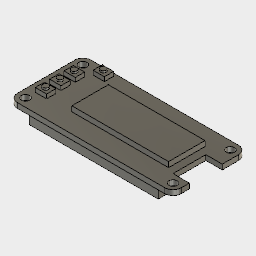
2900 Feather OLED Wing (Autodesk Fusion 360 design; units mm, degrees)
Autodesk Fusion 360 part; units mm, degrees
sketch "PCB" plane through (0, 0, 0) normal (0, 0, 1) x (1, 0, 0)
  line L0 (0, 0) -> (50.8, 0)
  line L1 (50.8, 0) -> (50.8, 22.86)
  line L2 (50.8, 22.86) -> (0, 22.86)
  line L3 (0, 22.86) -> (0, 0)
  circle A0 centre (2.54, 2.54) radius 1.27
  line L4 (0, 11.43) -> (51, 11.43) construction
  circle A1 centre (2.54, 20.32) radius 1.27
  line L5 (25.4, 22.86) -> (25.4, 0) construction
  circle A2 centre (48.26, 20.32) radius 1.27
  circle A3 centre (48.26, 2.54) radius 1.27
  line L6 (45.72, 15.24) -> (50.8, 15.24)
  line L7 (50.8, 15.24) -> (50.8, 5.08)
  line L8 (50.8, 5.08) -> (45.72, 5.08)
  line L9 (45.72, 5.08) -> (45.72, 15.24)
  dimension "d1" = 50.8
  dimension "d2" = 22.86
  dimension "d3" = 2.54
  dimension "d4" = 2.54
  dimension "d5" = 2.54
  dimension "d9" = 5.08
  dimension "d10" = 10.16
  dimension "d11" = 5.08
  measures "d1" distance of L0.start L0.end
  measures "d2" distance of L0.start L2.end
  measures "d3" diameter of A0
  measures "d4" distance of L0 A0.centre
  measures "d5" distance of L3 A0.centre
  measures "d9" distance of L6.start L6.end
  measures "d10" distance of L6.start L8.end
  measures "d11" distance of L0 L8
extrude "Extrude1" add sketch "PCB" against normal blind 1.6 contours L0 L1 L2 L3 L6 L8 L9 makes body 1
fillet "Fillet1" radius 2.54 4 edges at (0, 22.86, -0.8) (0, 0, -0.8) (50.8, 0, -0.8) (50.8, 22.86, -0.8) on bodies 1
sketch "OLED" plane through (0, 0, 0) normal (0, 0, 1) x (-1, 0, 0)
  circle A0 centre (-2.54, -2.54) radius 1.27
  circle A1 centre (-2.54, -20.32) radius 1.27
  circle A2 centre (-48.26, -2.54) radius 1.27
  circle A3 centre (-48.26, -20.32) radius 1.27
  arc A4 (-50.8, -20.32) -> (-48.26, -22.86) centre (-48.26, -20.32) ccw
  line L0 (-48.26, -22.86) -> (-2.54, -22.86)
  arc A5 (-2.54, -22.86) -> (0, -20.32) centre (-2.54, -20.32) ccw
  line L1 (0, -20.32) -> (0, -2.54)
  arc A6 (0, -2.54) -> (-2.54, 0) centre (-2.54, -2.54) ccw
  line L2 (-2.54, 0) -> (-48.26, 0)
  arc A7 (-48.26, 0) -> (-50.8, -2.54) centre (-48.26, -2.54) ccw
  line L3 (-50.8, -2.54) -> (-50.8, -5.08)
  line L4 (-50.8, -5.08) -> (-45.72, -5.08)
  line L5 (-45.72, -5.08) -> (-45.72, -15.24)
  line L6 (-45.72, -15.24) -> (-50.8, -15.24)
  line L7 (-50.8, -15.24) -> (-50.8, -20.32)
  line L8 (-13.46, -17.27) -> (-43.43, -17.27)
  line L9 (-43.43, -17.27) -> (-43.43, -5.97)
  line L10 (-43.43, -5.97) -> (-13.46, -5.97)
  line L11 (-13.46, -5.97) -> (-13.46, -17.27)
  dimension "d12" = 29.97
  dimension "d13" = 11.3
  dimension "d14" = 5.97
  dimension "d15" = 13.46
  measures "d12" distance of L9.end L10.end
  measures "d13" distance of L8.start L10.end
  measures "d14" distance of L2 L10
  measures "d15" distance of L1 L11
extrude "Extrude2" add sketch "OLED" along normal blind 1.62 separate body contours L8 L9 L10 L11 makes body 2
sketch "buttons" plane through (0, 0, 0) normal (0, 0, 1) x (-1, 0, 0)
  circle A0 centre (-2.54, -2.54) radius 1.27
  circle A1 centre (-2.54, -20.32) radius 1.27
  circle A2 centre (-48.26, -2.54) radius 1.27
  circle A3 centre (-48.26, -20.32) radius 1.27
  arc A4 (-50.8, -20.32) -> (-48.26, -22.86) centre (-48.26, -20.32) ccw
  line L0 (-48.26, -22.86) -> (-2.54, -22.86)
  arc A5 (-2.54, -22.86) -> (0, -20.32) centre (-2.54, -20.32) ccw
  line L1 (0, -20.32) -> (0, -2.54)
  arc A6 (0, -2.54) -> (-2.54, 0) centre (-2.54, -2.54) ccw
  line L2 (-2.54, 0) -> (-48.26, 0)
  arc A7 (-48.26, 0) -> (-50.8, -2.54) centre (-48.26, -2.54) ccw
  line L3 (-50.8, -2.54) -> (-50.8, -5.08)
  line L4 (-50.8, -5.08) -> (-45.72, -5.08)
  line L5 (-45.72, -5.08) -> (-45.72, -15.24)
  line L6 (-45.72, -15.24) -> (-50.8, -15.24)
  line L7 (-50.8, -15.24) -> (-50.8, -20.32)
  line L8 (-6.068, -5.535) -> (-2.568, -5.535)
  line L9 (-2.568, -5.535) -> (-2.568, -8.435)
  line L10 (-2.568, -8.435) -> (-6.068, -8.435)
  line L11 (-6.068, -8.435) -> (-6.068, -5.535)
  line L12 (-6.068, -5.535) -> (-2.568, -8.435) construction
  line L13 (-2.568, -5.535) -> (-6.068, -8.435) construction
  line L14 (-6.068, -9.98) -> (-2.568, -9.98)
  line L15 (-2.568, -9.98) -> (-2.568, -12.88)
  line L16 (-2.568, -12.88) -> (-6.068, -12.88)
  line L17 (-6.068, -12.88) -> (-6.068, -9.98)
  line L18 (-6.068, -9.98) -> (-2.568, -12.88) construction
  line L19 (-2.568, -9.98) -> (-6.068, -12.88) construction
  line L20 (-6.068, -14.425) -> (-2.568, -14.425)
  line L21 (-2.568, -14.425) -> (-2.568, -17.325)
  line L22 (-2.568, -17.325) -> (-6.068, -17.325)
  line L23 (-6.068, -17.325) -> (-6.068, -14.425)
  line L24 (-6.068, -14.425) -> (-2.568, -17.325) construction
  line L25 (-2.568, -14.425) -> (-6.068, -17.325) construction
  line L26 (-10.386, -19.124) -> (-6.886, -19.124)
  line L27 (-6.886, -19.124) -> (-6.886, -22.024)
  line L28 (-6.886, -22.024) -> (-10.386, -22.024)
  line L29 (-10.386, -22.024) -> (-10.386, -19.124)
  line L30 (-10.386, -19.124) -> (-6.886, -22.024) construction
  line L31 (-6.886, -19.124) -> (-10.386, -22.024) construction
  point P0 (-4.318, -6.985)
  point P1 (-4.318, -11.43)
  point P2 (-4.318, -15.875)
  point P3 (-8.636, -20.574)
  dimension "d18" = 3.5
  dimension "d19" = 2.9
  dimension "d20" = 4.318
  dimension "d21" = 6.985
  dimension "d22" = 3.5
  dimension "d23" = 2.9
  dimension "d24" = 4.318
  dimension "d25" = 11.43
  dimension "d26" = 3.5
  dimension "d27" = 2.9
  dimension "d28" = 4.318
  dimension "d29" = 15.875
  dimension "d37" = 3.5
  dimension "d38" = 2.9
  dimension "d39" = 8.636
  dimension "d41" = 20.574
  measures "d18" distance of L9.end L10.end
  measures "d19" distance of L8.end L9.end
  measures "d20" distance of L1 P0
  measures "d21" distance of L2 P0
  measures "d22" distance of L15.end L16.end
  measures "d23" distance of L14.end L15.end
  measures "d24" distance of L1 P1
  measures "d25" distance of L2 P1
  measures "d26" distance of L21.end L22.end
  measures "d27" distance of L20.end L21.end
  measures "d28" distance of L1 P2
  measures "d29" distance of L2 P2
  measures "d37" distance of L27.end L28.end
  measures "d38" distance of L26.end L27.end
  measures "d39" distance of L1 P3
  measures "d41" distance of L2 P3
extrude "Extrude3" add sketch "buttons" along normal blind 1.3 contours L8 L9 L10 L11 | L14 L15 L16 L17 | L20 L21 L22 L23 | L26 L27 L28 L29 bodies 1
sketch "button actuators" plane through (0, 0, 1.3) normal (0, 0, 1) x (-1, 0, 0)
  line L0 (-6.068, -17.325) -> (-2.568, -17.325)
  line L1 (-2.568, -17.325) -> (-2.568, -14.425)
  line L2 (-2.568, -14.425) -> (-6.068, -14.425)
  line L3 (-6.068, -14.425) -> (-6.068, -17.325)
  circle A0 centre (-4.318, -15.875) radius 0.85
  line L4 (-6.068, -12.88) -> (-2.568, -12.88)
  line L5 (-2.568, -12.88) -> (-2.568, -9.98)
  line L6 (-2.568, -9.98) -> (-6.068, -9.98)
  line L7 (-6.068, -9.98) -> (-6.068, -12.88)
  line L8 (-6.068, -8.435) -> (-2.568, -8.435)
  line L9 (-2.568, -8.435) -> (-2.568, -5.535)
  line L10 (-2.568, -5.535) -> (-6.068, -5.535)
  line L11 (-6.068, -5.535) -> (-6.068, -8.435)
  circle A1 centre (-4.318, -11.43) radius 0.85
  circle A2 centre (-4.318, -6.985) radius 0.85
  line L12 (-10.386, -22.024) -> (-6.886, -22.024)
  line L13 (-6.886, -22.024) -> (-6.886, -19.124)
  line L14 (-6.886, -19.124) -> (-10.386, -19.124)
  line L15 (-10.386, -19.124) -> (-10.386, -22.024)
  circle A3 centre (-8.636, -20.574) radius 0.85
  point P0 (-8.636, -20.574)
  dimension "d32" = 1.7
  dimension "d33" = 1.7
  dimension "d34" = 1.7
  dimension "d42" = 1.7
  measures "d32" diameter of A0
  measures "d33" diameter of A1
  measures "d34" diameter of A2
  measures "d42" diameter of A3
extrude "Extrude4" add sketch "button actuators" along normal blind 0.6 contours A0 | A1 | A2 | A3 bodies 1
sketch "header strips" plane through (0, 0, -1.6) normal (0, 0, -1) x (1, 0, 0)
  arc A0 (48.26, -22.86) -> (50.8, -20.32) centre (48.26, -20.32) ccw
  line L0 (50.8, -20.32) -> (50.8, -15.24)
  line L1 (50.8, -15.24) -> (45.72, -15.24)
  line L2 (45.72, -15.24) -> (45.72, -5.08)
  line L3 (45.72, -5.08) -> (50.8, -5.08)
  line L4 (50.8, -5.08) -> (50.8, -2.54)
  arc A1 (50.8, -2.54) -> (48.26, 0) centre (48.26, -2.54) ccw
  line L5 (48.26, 0) -> (2.54, 0)
  arc A2 (2.54, 0) -> (0, -2.54) centre (2.54, -2.54) ccw
  line L6 (0, -2.54) -> (0, -20.32)
  arc A3 (0, -20.32) -> (2.54, -22.86) centre (2.54, -20.32) ccw
  line L7 (2.54, -22.86) -> (48.26, -22.86)
  circle A4 centre (2.54, -2.54) radius 1.27
  circle A5 centre (2.54, -20.32) radius 1.27
  circle A6 centre (48.26, -2.54) radius 1.27
  circle A7 centre (48.26, -20.32) radius 1.27
  line L8 (6.2, 0) -> (46.2, 0)
  line L9 (46.2, 0) -> (46.2, -2.5)
  line L10 (46.2, -2.5) -> (6.2, -2.5)
  line L11 (6.2, -2.5) -> (6.2, 0)
  line L12 (15.2, -22.86) -> (46.2, -22.86)
  line L13 (46.2, -22.86) -> (46.2, -20.36)
  line L14 (46.2, -20.36) -> (15.2, -20.36)
  line L15 (15.2, -20.36) -> (15.2, -22.86)
  dimension "d43" = 40
  dimension "d44" = 2.5
  dimension "d46" = 31
  dimension "d47" = 2.5
  dimension "d51" = 4.6
  dimension "d52" = 4.6
  measures "d43" distance of L8.start L8.end
  measures "d44" distance of L8.start L10.end
  measures "d46" distance of L12.start L12.end
  measures "d47" distance of L12.start L14.end
  measures "d51" distance of L4 L9
  measures "d52" distance of L0 L13
extrude "Extrude5" add sketch "header strips" along normal blind 2.5 separate body contours L7 L12 L13 L14 L15 | L5 L8 L9 L10 L11 makes body 3 at (32.8667, 0, -2.4333) makes body 4 at (35.8667, 22.0267, -1.6)
named bodies: "PCB", "OLED", "header A", "header B"
